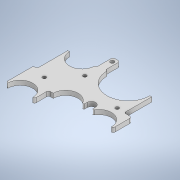
# Autodesk Inventor part: Bottle layout pt2
Saved by Autodesk Inventor 2021 (Build 250183000, 183)
## iProperties
Created: 2020-07-28
Part Number: Bottle layout pt2
Material: Generic
Document SubType Name: Modeling
Designer: jgray
Density: 1 g/cm^3
Appearance: Default
Author: jgray
Autodesk Inventor part; units mm, degrees
ref_plane "YZ Plane" through (0, 0, 0) normal (1, 0, 0) x (0, 1, 0)
ref_plane "XZ Plane" through (0, 0, 0) normal (0, 1, 0) x (-1, 0, 0)
ref_plane "XY Plane" through (0, 0, 0) normal (0, 0, 1) x (1, 0, 0)
sketch "Sketch1" plane through (0, 0, 0) normal (0, 1, 0) x (-1, 0, 0)
  line L0 (-56.25, 58.25) -> (56.25, 58.25)
  line L1 (56.25, 58.25) -> (56.25, -58.25)
  line L2 (56.25, -58.25) -> (-56.25, -58.25)
  line L3 (-56.25, -58.25) -> (-56.25, 58.25)
  line L4 (-56.25, 58.25) -> (56.25, -58.25) construction
  line L5 (56.25, 58.25) -> (-56.25, -58.25) construction
  point P0 (0, 0)
  dimension "d0" = 112.5
  dimension "d1" = 116.5
  constraints: 12 end point, 2 midpoint, 2 parallel, 1 horizontal, 1 perpendicular
  measures "d0" distance of L1.end L2.end
  measures "d1" distance of L0.end L1.end
extrude "Extrusion1" add sketch "Sketch1" along normal blind 5
sketch "Sketch2" plane through (0, 5, 0) normal (0, 1, 0) x (1, 0, 0)
  circle A0 centre (18.5, 28) radius 23.85
  circle A1 centre (37, -23.25) radius 13.85
  circle A2 centre (-35, -38.75) radius 13.85
  circle A3 centre (-30.9, 25.8) radius 13.85
  circle A4 centre (0, -23.25) radius 13.85
  line L0 (56.25, 58.25) -> (-56.25, 58.25) projected
  line L1 (-56.25, -58.25) -> (56.25, -58.25) projected
  line L2 (0, -105.9299) -> (0, 123.2086) construction
  line L3 (-76.4777, -38.75) -> (-5.35, -38.75) construction
  line L4 (-123.5447, -23.25) -> (82.5572, -23.25) construction
  line L5 (56.25, -58.25) -> (56.25, 58.25) construction
  point P0 (0, 0)
  dimension "d4" = 47.7
  dimension "d5" = 27.7
  dimension "d6" = 27.7
  dimension "d7" = 27.7
  dimension "d8" = 27.7
  dimension "d9" = 116.5
  dimension "d10" = 112.5
  dimension "d13" = 37
  dimension "d14" = 18.5
  dimension "d15" = 30.9
  dimension "d18" = 19.5
  dimension "d19" = 35
  dimension "d20" = 35
  dimension "d42" = 25.8
  dimension "d43" = 28
  constraints: 6 end point, 5 centre point, 5 point on line, 1 horizontal, 1 perpendicular, 1 vertical
  measures "d4" diameter of A0
  measures "d5" diameter of A1
  measures "d6" diameter of A2
  measures "d7" diameter of A3
  measures "d8" diameter of A4
  measures "d9" distance between parallel lines of L0 L1
  measures "d10" distance of L1.start L1.end
  measures "d13" distance of A4.centre A1.centre
  measures "d14" distance from line of A0.centre L2
  measures "d15" distance from line of A3.centre L2
  measures "d18" distance between parallel lines of L1 L3
  measures "d19" distance between parallel lines of L1 L4
  measures "d20" horizontal distance of A2.centre A4.centre
  measures "d42" vertical distance of point (0, 0) A3.centre
  measures "d43" vertical distance of point (0, 0) A0.centre
extrude "Extrusion2" cut sketch "Sketch2" against normal blind 5
sketch "Sketch5" plane through (0, 5, 0) normal (0, 1, 0) x (1, 0, 0)
  line L0 (-56.25, 58.25) -> (-56.25, -58.25) construction
  circle A0 centre (0, -23.25) radius 13.85 construction
  circle A1 centre (37, -23.25) radius 13.85 construction
  circle A2 centre (-30.9, 25.8) radius 13.85 construction
  line L1 (56.25, 58.25) -> (-56.25, 58.25) construction
  line L2 (-17.15, -23.25) -> (-13.85, -23.25) construction
  line L3 (-46.75, -8.1822) -> (-46.85, -8.1822)
  line L4 (-13.85, -23.25) -> (-17.15, -23.25)
  line L5 (56.25, -58.25) -> (56.25, 58.25)
  line L6 (-46.85, -8.1822) -> (-46.75, -8.1822)
  arc A3 (-13.85, -23.25) -> (13.85, -23.25) centre (0, -23.25) ccw
  arc A4 (23.15, -23.25) -> (50.85, -23.25) centre (37, -23.25) ccw
  line L7 (-44.75, 58.25) -> (42.35, 58.25)
  line L8 (-48.85, -38.75) -> (-48.85, -38.75)
  line L9 (-50.85, -36.75) -> (-50.85, -10.1822)
  line L10 (-48.85, -8.1822) -> (-48.75, -8.1822)
  arc A5 (-50.85, -36.75) -> (-48.85, -38.75) centre (-48.85, -36.75) ccw
  arc A6 (-48.85, -8.1822) -> (-50.85, -10.1822) centre (-48.85, -10.1822) ccw
  line L11 (50.85, -23.25) -> (50.85, -23.25)
  line L12 (52.85, -21.25) -> (52.85, -4.75)
  line L13 (50.85, -2.75) -> (46.35, -2.75)
  arc A7 (50.85, -23.25) -> (52.85, -21.25) centre (50.85, -21.25) ccw
  arc A8 (52.85, -4.75) -> (50.85, -2.75) centre (50.85, -4.75) ccw
  line L14 (-44.7516, 25.8) -> (-44.7516, 25.8)
  line L15 (-46.75, 28.0339) -> (-46.75, 58.25)
  line L16 (-44.75, 58.25) -> (-46.75, 58.25)
  line L17 (-17.0566, 26.2282) -> (-17.0566, 26.2282)
  line L18 (-15.05, 27.8) -> (-15.05, 42.25)
  line L19 (-5.35, 27.98) -> (-5.35, 27.98)
  line L20 (-7.35, 30.25) -> (-7.35, 42.25)
  line L21 (42.35, 27.98) -> (42.35, 27.98)
  line L22 (44.35, 58.25) -> (42.35, 58.25)
  circle A9 centre (0, -23.25) radius 13.85
  circle A10 centre (37, -23.25) radius 13.85
  line L23 (44.35, 58.25) -> (44.35, -0.75)
  line L24 (42.35, 27.98) -> (44.35, 27.98)
  line L25 (-5.35, 27.98) -> (-5.35, 27.98)
  line L26 (-7.35, 29.98) -> (-7.35, 30.25)
  line L27 (-17.0566, 26.2282) -> (-17.0566, 26.2282)
  line L28 (-15.05, 28.0029) -> (-15.05, 28.0029)
  line L29 (-46.75, 28.0339) -> (-46.75, -6.1822)
  arc A11 (-48.75, -8.1822) -> (-46.75, -6.1822) centre (-48.75, -6.1822) ccw
  line L30 (-44.75, 25.8) -> (-46.75, 25.8)
  line L31 (-21.15, -38.75) -> (-21.15, -38.75)
  line L32 (-19.15, -36.75) -> (-19.15, -25.25)
  arc A12 (-21.15, -38.75) -> (-19.15, -36.75) centre (-21.15, -36.75) ccw
  arc A13 (-17.15, -23.25) -> (-19.15, -25.25) centre (-17.15, -25.25) ccw
  line L33 (-17.05, 25.8) -> (-17.05, 25.8)
  arc A14 (-17.05, 25.8) -> (-15.05, 27.8) centre (-17.05, 27.8) ccw
  line L34 (-56.25, -58.25) -> (56.25, -58.25)
  line L35 (56.25, -58.25) -> (56.25, 58.25)
  line L36 (56.25, 58.25) -> (-56.25, 58.25)
  line L37 (-56.25, 58.25) -> (-56.25, -58.25)
  circle A15 centre (-30.9, 25.8) radius 13.85 projected
  circle A16 centre (-30.9, 25.8) radius 13.85
  line L38 (13.85, -23.25) -> (13.85, -13.25)
  circle A17 centre (0, -23.25) radius 13.85 projected
  line L39 (23.15, -23.25) -> (23.15, -13.25)
  circle A18 centre (37, -23.25) radius 13.85 projected
  arc A19 (23.15, -13.25) -> (13.85, -13.25) centre (18.5, -13.25) ccw
  circle A20 centre (18.5, 28) radius 23.85
  circle A21 centre (18.5, 28) radius 23.85 projected
  line L40 (56.25, 58.25) -> (-56.25, 58.25) projected
  circle A22 centre (-35, -38.75) radius 13.85
  circle A23 centre (-35, -38.75) radius 13.85 projected
  arc A24 (44.35, -0.75) -> (46.35, -2.75) centre (46.35, -0.75) ccw
  line L41 (-5.35, 27.98) -> (-5.35, 27.98)
  arc A25 (-7.35, 29.98) -> (-5.35, 27.98) centre (-5.35, 29.98) ccw
  line L42 (-13.05, 44.25) -> (-9.35, 44.25)
  arc A26 (-13.05, 44.25) -> (-15.05, 42.25) centre (-13.05, 42.25) ccw
  arc A27 (-7.35, 42.25) -> (-9.35, 44.25) centre (-9.35, 42.25) ccw
  point P0 (0, 0)
  point P1 (0, 0)
  point P2 (44.35, -2.75)
  point P3 (-50.85, -38.75)
  point P4 (52.85, -23.25)
  point P5 (-15.05, 58.25)
  point P6 (-7.35, 58.25)
  point P7 (-48.85, -40.25)
  point P8 (50.85, -23.25)
  point P9 (-21.15, -40.25)
  point P10 (50.85, -23.25)
  point P11 (-7.35, 58.25)
  point P12 (50.85, -23.25)
  point P13 (-17.05, 25.8)
  point P14 (-7.35, 27.98)
  point P15 (-7.35, 29.98)
  point P16 (-21.15, -38.75)
  point P17 (-48.85, -38.75)
  dimension "d53" = 27.7
  dimension "d54" = 27.7
  dimension "d26" = 2
  dimension "d27" = 2
  dimension "d28" = 2
  dimension "d29" = 2
  dimension "d30" = 2
  dimension "d32" = 2
  dimension "d33" = 2
  dimension "d34" = 2
  dimension "d35" = 2
  dimension "d38" = 27.7
  dimension "d39" = 10
  dimension "d40" = 10
  dimension "d45" = 25.8
  dimension "d46" = 23.25
  dimension "d47" = 23.25
  dimension "d50" = 37
  dimension "d56" = 19.15
  dimension "d57" = 50.85
  dimension "d58" = 46.75
  dimension "d59" = 2
  dimension "d60" = 6.1822
  dimension "d61" = 31.7
  dimension "d63" = 30.9
  dimension "d64" = 3.4
  dimension "d65" = 11.9
  dimension "d66" = 61
  dimension "d67" = 47.7
  dimension "d68" = 28
  dimension "d69" = 18.5
  dimension "d71" = 30.27
  dimension "d72" = 27.7
  dimension "d73" = 2
  dimension "d74" = 30.27
  dimension "d75" = 2
  dimension "d76" = 112.5
  dimension "d77" = 116.5
  dimension "d79" = 14
  dimension "d80" = 2
  dimension "d81" = 51.7
  dimension "d82" = 2
  constraints: 84 end point, 40 point on circle, 30 tangent, 23 point on line, 20 centre point, 15 perpendicular, 9 horizontal, 5 coincident, 5 vertical, 3 equal radius, 3 parallel, 2 collinear, 2 concentric, 2 horizontal alignment, 1 line through centre, 1 midpoint, 11 other
  measures "d26" distance of L8.start point (-50.85, -38.75)
  measures "d27" radius of A5
  measures "d28" distance of L11.start point (52.85, -23.25)
  measures "d29" radius of A7
  measures "d30" distance from line of L21.end L23
  measures "d32" radius of A11
  measures "d33" radius of A12
  measures "d34" distance from line of L18 L33.start
  measures "d35" radius of A14
  measures "d38" diameter of A2
  measures "d39" distance of L38.start L38.end
  measures "d40" distance of L39.start L39.end
  measures "d45" vertical distance of point (0, 0) A2.centre
  measures "d46" vertical distance of point (0, 0) A1.centre
  measures "d47" distance of point (0, 0) A0.centre
  measures "d50" horizontal distance of A1.centre point (0, 0)
  measures "d56" distance from line of L32 point (0, 0)
  measures "d57" distance from line of L9 point (0, 0)
  measures "d58" distance from line of L29 point (0, 0)
  measures "d59" radius of A6
  measures "d60" vertical distance of point (0, 0) A11.centre
  measures "d61" distance between parallel lines of L18 L15
  measures "d63" horizontal distance of point (0, 0) A15.centre
  measures "d64" distance between parallel lines of L5 L12
  measures "d65" distance between parallel lines of L5 L23
  measures "d66" distance between parallel lines of L1 L13
  measures "d67" diameter of A20
  measures "d68" vertical distance of point (0, 0) A21.centre
  measures "d69" horizontal distance of A21.centre point (0, 0)
  measures "d71" distance between parallel lines of L7 L24
  measures "d72" diameter of A22
  measures "d73" radius of A24
  measures "d74" distance of point (-7.35, 58.25) point (-7.35, 27.98)
  measures "d75" radius of A25
  measures "d76" distance between parallel lines of L35 L0
  measures "d77" distance between parallel lines of L36 L34
  measures "d79" distance between parallel lines of L7 L42
  measures "d80" radius of A26
  measures "d81" distance between parallel lines of L23 L20
  measures "d82" radius of A27
extrude "Extrusion3" cut sketch "Sketch5" against normal blind 10 contours A3 L38 A19 L39 A4 A7 L12 A8 L13 A24 L23 L36 L5 L34 L37 L15 L29 A11 L10 A6 L9 A5 A22 A12 L32 A13 L4 | L29 L15 L16 L7 L22 L23 L24 A20 A25 L26 L20 A27 L42 A26 L18 A14 A15 L30
fillet "Fillet2" radius 1 2 edges at (13.85, 2.5, 23.25) (23.15, 2.5, 23.25)
sketch "Sketch7" plane through (0, 5, 0) normal (0, 1, 0) x (1, 0, 0)
  line L0 (-7.35, 29.98) -> (-7.35, 42.25) projected
  line L1 (-9.35, 44.25) -> (-13.05, 44.25) projected
  point P0 (0, 0)
  point P1 (-34, -13)
  point P2 (-13, 11)
  point P3 (36, -2)
  point P4 (-11.2, 39.75)
  dimension "d83" = 13
  dimension "d84" = 34
  dimension "d85" = 36
  dimension "d86" = 2
  dimension "d87" = 11
  dimension "d88" = 13
  dimension "d96" = 3.85
  dimension "d97" = 4.5
  measures "d83" horizontal distance of point (-13, 11) point (0, 0)
  measures "d84" horizontal distance of point (-34, -13) point (0, 0)
  measures "d85" horizontal distance of point (36, -2) point (0, 0)
  measures "d86" vertical distance of point (36, -2) point (0, 0)
  measures "d87" vertical distance of point (-13, 11) point (0, 0)
  measures "d88" vertical distance of point (-34, -13) point (0, 0)
  measures "d96" distance from line of L0 point (-11.2, 39.75)
  measures "d97" distance from line of L1 point (-11.2, 39.75)
hole "Hole1" at (-34, 5, 13) at (-13, 5, -11) at (36, 5, 2) direction (0, -1, 0) diameter 3.8 end through all
hole "Hole2" at (-11.2, 5, -39.75) direction (0, -1, 0) diameter 4.2 end through all
body "Solid1"
